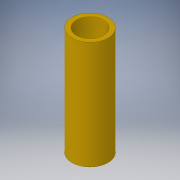
# Autodesk Inventor part: Abstandshalter 12mm
Saved by Autodesk Inventor 2018 (Build 220112000, 112)
## iProperties
Created: 2019-03-05
Part Number: Abstandshalter 12mm
Material: ABS-Kunststoff
Document SubType Name: Modeling
Designer: RedBots
Density: 1.06 g/cm^3
Appearance: Glatt - schwarz
Mass: 0.0699319 g
Surface Area: 2.74889 cm^2
Volume: 0.0659734 cm^3
Author: RedBots
Autodesk Inventor part; units mm, degrees
ref_plane "YZ Plane" through (0, 0, 0) normal (1, 0, 0) x (0, 1, 0)
ref_plane "XZ Plane" through (0, 0, 0) normal (0, 1, 0) x (-1, 0, 0)
ref_plane "XY Plane" through (0, 0, 0) normal (0, 0, 1) x (1, 0, 0)
sketch "Skizze1" plane through (0, 0, 0) normal (0, 0, 1) x (1, 0, 0)
  circle A0 centre (0, 0) radius 1.5
  circle A1 centre (0, 0) radius 2
  dimension "d0" = 3
  dimension "d1" = 4
  constraints: 2 centre point, 2 coincident
  measures "d0" diameter of A0
  measures "d1" diameter of A1
extrude "Extrusion1" add sketch "Skizze1" along normal blind 12
